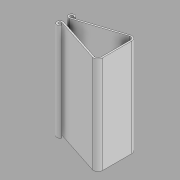
# Autodesk Inventor part: Assignment 2
Saved by Autodesk Inventor 2022 (Build 260153000, 153)
## iProperties
Created: 2021-09-20
Part Number: Assignment 2
Material: Generic
Document SubType Name: Modeling
Designer: seang
Density: 1 g/cm^3
Appearance: Default
Author: seang
Autodesk Inventor part; units mm, degrees
ref_plane "YZ Plane" through (0, 0, 0) normal (1, 0, 0) x (0, 1, 0)
ref_plane "XZ Plane" through (0, 0, 0) normal (0, 1, 0) x (-1, 0, 0)
ref_plane "XY Plane" through (0, 0, 0) normal (0, 0, 1) x (1, 0, 0)
sketch "Sketch1" plane through (0, 0, 0) normal (0, 1, 0) x (-1, 0, 0)
  line L0 (0, 0) -> (6, 0) construction
  line L1 (0, 0) -> (0, -4.8109)
  line L2 (0.5522, -6.0201) -> (1.6839, -6.0201) construction
  line L3 (0, -6) -> (3.6357, -6) construction
  arc A0 (0, -4.8109) -> (1.1715, -5.7961) centre (1, -4.8109) ccw
  line L4 (1.1715, -5.7961) -> (16.0448, -0.9635)
  line L5 (1.1715, -5.7961) -> (19.9281, -5.7961) construction
  line L6 (16.3387, 0) -> (18.0887, 0) construction
  arc A1 (15.4028, -2.2235) -> (16.0448, -0.9635) centre (16.3539, -1.9145) ccw
  line L7 (0, 0) -> (0, 4.8109)
  arc A2 (1.1715, 5.7961) -> (0, 4.8109) centre (1, 4.8109) ccw
  line L8 (1.1715, 5.7961) -> (16.0448, 0.9635)
  arc A3 (16.0448, 0.9635) -> (15.4028, 2.2235) centre (16.3539, 1.9145) ccw
  line L9 (16.1993, 1.439) -> (1.2956, 6.2815)
  arc A4 (1.2956, 6.2815) -> (-0.5, 4.8109) centre (1, 4.8109) ccw
  line L10 (-0.5, 4.8109) -> (-0.5, 0)
  line L11 (16.1993, -1.439) -> (1.2956, -6.2815)
  arc A5 (-0.5, -4.8109) -> (1.2956, -6.2815) centre (1, -4.8109) ccw
  line L12 (-0.5, -4.8109) -> (-0.5, 0)
  arc A6 (15.8783, -2.069) -> (16.1993, -1.439) centre (16.3539, -1.9145) ccw
  arc A7 (16.1993, 1.439) -> (15.8783, 2.069) centre (16.3539, 1.9145) ccw
  line L13 (15.8783, 2.069) -> (15.4028, 2.2235)
  line L14 (15.8783, -2.069) -> (15.4028, -2.2235)
  dimension "d3" = 6
  dimension "d16" = 1
  dimension "d17" = 18
  dimension "d28" = 0.5
  dimension "d29" = 0.5
  constraints: 30 end point, 16 point on circle, 8 centre point, 5 horizontal, 2 coincident, 2 tangent, 1 point on line, 1 vertical, 4 other
  measures "d3" distance of L0.start L3.start
  measures "d16" radius of A0
  measures "d17" angle of L5 L4
  measures "d28" distance between parallel lines of L8 L9
  measures "d29" distance between parallel lines of L4 L11
extrude "Extrusion1" add sketch "Sketch1" along normal blind 32
body "Solid1"
